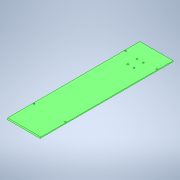
# Autodesk Inventor part: 前カバー中盤
Saved by Autodesk Inventor 2022 (Build 260153000, 153)
## iProperties
Created: 2022-11-07
Part Number: 前カバー中盤
Material: フェノール樹脂
Document SubType Name: Modeling
Designer: tdn82
Density: 1.38 g/cm^3
Appearance: 滑らか - 淡いオレンジ
Author: tdn82
Autodesk Inventor part; units mm, degrees
ref_plane "YZ Plane" through (0, 0, 0) normal (1, 0, 0) x (0, 1, 0)
ref_plane "XZ Plane" through (0, 0, 0) normal (0, 1, 0) x (-1, 0, 0)
ref_plane "XY Plane" through (0, 0, 0) normal (0, 0, 1) x (1, 0, 0)
sketch "スケッチ1" plane through (0, 0, 0) normal (0, 1, 0) x (-1, 0, 0)
  line L0 (0, 0) -> (-80, 0)
  line L1 (-80, 0) -> (-80, -320)
  line L2 (-80, -320) -> (0, -320)
  line L3 (0, -320) -> (0, 0)
  dimension "d0" = 320
  dimension "d1" = 80
  constraints: 8 end point, 2 parallel, 1 horizontal, 1 perpendicular
  measures "d0" distance of L2.end L0.start
  measures "d1" distance of L0.start L0.end
extrude "押し出し1" add sketch "スケッチ1" along normal blind 2
sketch "スケッチ3" plane through (0, 0, 0) normal (0, -1, 0) x (1, 0, 0)
  line L0 (80, -320) -> (0, -320) projected
  line L1 (80, 0) -> (80, -320) projected
  point P0 (0, 0)
  point P1 (48, -280)
  point P2 (33, -280)
  point P3 (48, -258)
  point P4 (33, -258)
  dimension "d20" = 40
  dimension "d21" = 32
  dimension "d24" = 15
  dimension "d27" = 22
  constraints: 1 horizontal, 1 vertical, 3 other
  measures "d20" distance from line of L0 point (48, -280)
  measures "d21" distance from line of point (48, -280) L1
  measures "d24" distance of point (48, -280) point (33, -280)
  measures "d27" distance of point (48, -280) point (48, -258)
hole "穴1" at (48, 0, -280) at (33, 0, -280) at (48, 0, -258) at (33, 0, -258) direction (0, 1, 0) diameter 3.2 end through all
chamfer "面取り2" distance 2 angle 45 1 edges at (40, 2, 0)
sketch "スケッチ5" plane through (0, 0, 0) normal (0, -1, 0) x (1, 0, 0)
  line L0 (80, 0) -> (80, -320) projected
  line L1 (0, 0) -> (80, 0) projected
  line L2 (0, -320) -> (0, 0) projected
  point P0 (77.5, -63)
  point P1 (77.5, -283)
  point P2 (2.5, -63)
  point P3 (2.5, -283)
  dimension "d43" = 2.5
  dimension "d44" = 63
  dimension "d45" = 220
  dimension "d53" = 2.5
  dimension "d54" = 63
  dimension "d55" = 220
  measures "d43" distance from line of point (77.5, -63) L0
  measures "d44" distance from line of point (77.5, -63) L1
  measures "d45" distance of point (77.5, -283) point (77.5, -63)
  measures "d53" distance from line of L2 point (2.5, -63)
  measures "d54" distance from line of L1 point (2.5, -63)
  measures "d55" distance of point (2.5, -63) point (2.5, -283)
hole "穴2" at (77.5, 0, -63) at (77.5, 0, -283) at (2.5, 0, -63) at (2.5, 0, -283) direction (0, 1, 0) diameter 3.2 end through all
